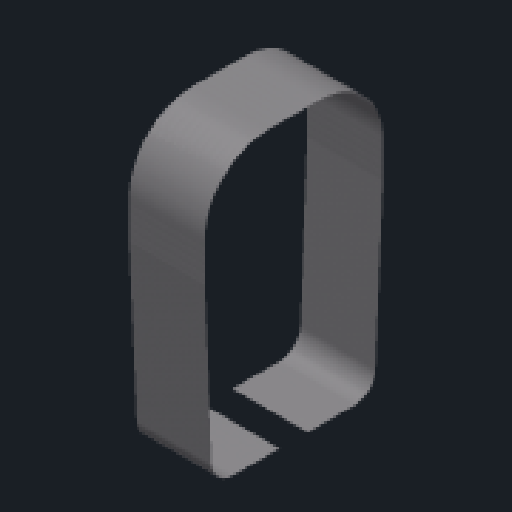
# Autodesk Inventor part: CARCASA_ALUM_1
Saved by Autodesk Inventor 2024.3 (Build 283343000, 343)
## iProperties
Created: 2024-05-14
Part Number: CARCASA_ALUM_1
Material: Steel, Mild, Welded
Document SubType Name: Sheet Metal
Designer: Niler
Density: 7.85 g/cm^3
Sheet Metal Rule: Default_mm
Appearance: Weld - Steel Mild
Flat Pattern Width: 45 cm
Flat Pattern Length: 428.336 cm
Flat Pattern Area: 19275.1 cm^2
Sheet Metal Width: 450.000 mm
Sheet Metal Length: 4283.362 mm
Sheet Metal Area: 1927512.891 mm^2
Author: Niler
Autodesk Inventor part; units mm, degrees
ref_plane "YZ Plane" through (0, 0, 0) normal (1, 0, 0) x (0, 1, 0)
ref_plane "XZ Plane" through (0, 0, 0) normal (0, 1, 0) x (-1, 0, 0)
ref_plane "XY Plane" through (0, 0, 0) normal (0, 0, 1) x (1, 0, 0)
sketch "Sketch1" plane through (0, 0, 0) normal (0, 1, 0) x (-1, 0, 0)
  line L0 (-225, 150) -> (225, 150)
  line L1 (225, 150) -> (225, -150)
  line L2 (225, -150) -> (-225, -150)
  line L3 (-225, -150) -> (-225, 150)
  line L4 (-225, 150) -> (225, -150) construction
  line L5 (225, 150) -> (-225, -150) construction
  point P0 (0, 0)
  dimension "d0" = 300
  dimension "d1" = 450
extrude "Plate1" add sketch "Sketch1" along normal blind 1.5
sketch "Sketch2" plane through (-225, -381.5, 531.5) normal (0, 0, 1) x (1, 0, 0)
  line L0 (450, 0) -> (0, 0)
  line L1 (0, 0) -> (0, -227)
  line L2 (0, -227) -> (450, -227)
  line L3 (450, -227) -> (450, 0)
  constraints: 6 end point, 1 horizontal, 1 perpendicular, 1 vertical
edge flange "Flange1" height 610 angle 90 thickness 1.5 bend radius 381.5 thickness toward (0, 0, 1) relief straight relief width 1.5 relief depth 0.75 corner gap 1.5 corner form 0 edges at (0, 0, 150) (0, 0, -150) wall of the first edge with corners at (225, -381.5, 531.5) (-225, -381.5, 531.5) (-225, -608.5, 531.5) (225, -608.5, 531.5)
bend "Bend1"
corner "Corner1"
sketch "Sketch3" plane through (-225, -608.5722, 531.4987) normal (0, -0.0361205, 0.9993474) x (1, 0, 0)
  line L0 (450, 0) -> (0, 0)
  line L1 (0, 0) -> (0, -960.9639)
  line L2 (0, -960.9639) -> (450, -960.9639)
  line L3 (450, -960.9639) -> (450, 0)
  constraints: 6 end point, 1 horizontal, 1 perpendicular, 1 vertical
edge flange "Flange2" height 961 angle 2.07 thickness 1.5 bend radius 2 thickness toward (0, -0.0361205, 0.9993474) relief straight relief width 1.5 relief depth 0.75 corner gap 1.5 corner form 0 edges at (0, -608.5, 531.5) (0, -608.5, -531.5) wall of the first edge with corners at (225, -608.5722, 531.4987) (-225, -608.5722, 531.4987) (-225, -1568.909, 496.7882) (225, -1568.909, 496.7882)
bend "Bend2"
corner "Corner2"
sketch "Sketch4" plane through (-225, -1685.1529, 376.3301) normal (0, -0.9999999, 0.0005236) x (1, 0, 0)
  line L0 (450, 0) -> (0, 0)
  line L1 (0, 0) -> (0, -17.2951)
  line L2 (0, -17.2951) -> (450, -17.2951)
  line L3 (450, -17.2951) -> (450, 0)
  constraints: 8 end point
edge flange "Flange3" height 135 angle 87.9 thickness 1.5 bend radius 120.6 thickness toward (0, -0.9999999, 0.0005236) relief straight relief width 1.5 relief depth 0.75 corner gap 1.5 corner form 0 edges at (0, -1568.909, 496.7882) (0, -1568.909, -496.7882) wall of the first edge with corners at (225, -1685.1529, 376.3301) (-225, -1685.1529, 376.3301) (-225, -1685.1619, 359.0349) (225, -1685.1619, 359.0349)
bend "Bend3"
corner "Corner3"
equation "\"d2\" = Thickness"
equation "\"d3\" = BendReliefWidth"
equation "\"d4\" = BendReliefDepth"
equation "\"d5\" = MinimumRemnant"
equation "\"d6\" = TransitionRadius"
equation "\"d10\" = CornerReliefSize"
equation "\"d11\" = GapSize"
equation "\"d12\" = JacobiRadiusSize"
equation "\"d13\" = BendReliefWidth"
equation "\"d14\" = BendReliefDepth"
equation "\"d15\" = MinimumRemnant"
equation "\"d16\" = TransitionRadius"
equation "\"d20\" = CornerReliefSize"
equation "\"d21\" = GapSize"
equation "\"d22\" = JacobiRadiusSize"
equation "\"d23\" = BendReliefWidth"
equation "\"d24\" = BendReliefDepth"
equation "\"d25\" = MinimumRemnant"
equation "\"d26\" = TransitionRadius"
equation "\"d30\" = CornerReliefSize"
equation "\"d31\" = GapSize"
equation "\"d32\" = JacobiRadiusSize"
equation "\"BendRadius\" = Thickness"
equation "\"BendReliefWidth\" = Thickness"
equation "\"BendReliefDepth\" = 0.5 * Thickness"
equation "\"CornerReliefSize\" = 4 * Thickness"
equation "\"MinimumRemnant\" = 2 * Thickness"
equation "\"TransitionRadius\" = BendRadius"
equation "\"JacobiRadiusSize\" = BendRadius"
equation "\"GapSize\" = Thickness"
equation "\"Thickness\" = 1.5"
body "Solid1"
